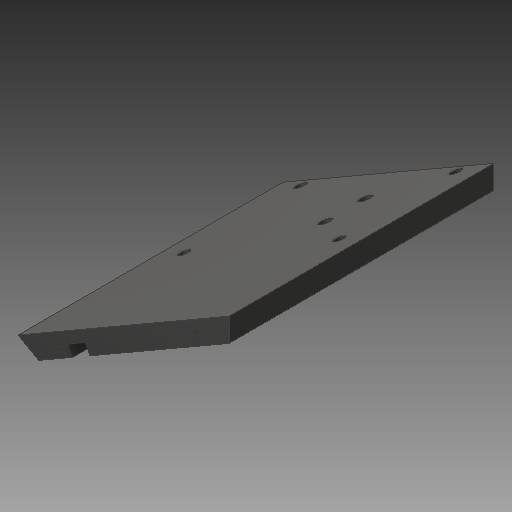
# Autodesk Inventor part: HB02
Saved by Autodesk Inventor 2017 (Build 210142000, 142)
## iProperties
Created: 2019-05-20
Part Number: HB02
Material: Polyethylene, High Density
Document SubType Name: Modeling
Designer: Dell
Density: 0.952 g/cm^3
Appearance: Smooth - Black
Mass: 1765.8 g
Surface Area: 2622.79 cm^2
Volume: 1854.83 cm^3
Author: Dell
Autodesk Inventor part; units mm, degrees
ref_plane "YZ Plane" through (0, 0, 0) normal (1, 0, 0) x (0, 1, 0)
ref_plane "XZ Plane" through (0, 0, 0) normal (0, 1, 0) x (-1, 0, 0)
ref_plane "XY Plane" through (0, 0, 0) normal (0, 0, 1) x (1, 0, 0)
sketch "Sketch1" plane through (0, 0, 0) normal (0, 0, 1) x (1, 0, 0)
  line L0 (262.89, 151.7796) -> (525.78, 0) construction
  line L1 (525.78, 0) -> (525.78, -303.5592) construction
  line L2 (525.78, -303.5592) -> (262.89, -455.3388) construction
  line L3 (262.89, -455.3388) -> (0, -303.5592) construction
  line L4 (0, -303.5592) -> (0, 0) construction
  line L5 (0, 0) -> (262.89, 151.7796)
  line L6 (0, 0) -> (25.4, -14.6647)
  line L7 (25.4, -14.6647) -> (262.89, 122.4502)
  line L8 (262.89, 122.4502) -> (262.89, 151.7796)
  point P0 (262.89, -151.7796)
  dimension "d0" = 525.78
  dimension "d2" = 25.4
  dimension "d3" = 60
  dimension "d4" = 60
  constraints: 18 end point, 1 coincident, 1 parallel, 1 vertical, 13 other
  measures "d0" distance between parallel lines of L1 L4
  measures "d2" distance between parallel lines of L5 L7
  measures "d3" angle of L5 L8
  measures "d4" angle of L5 L6
extrude "Extrusion1" add sketch "Sketch1" along normal blind 330.2
sketch "Sketch8" plane through (0, 0, 0) normal (0, 0, -1) x (-1, 0, 0)
  line L0 (-25.4, -14.6647) -> (-262.89, 122.4502) projected
  line L1 (-67.675, 9.7428) -> (-61.325, 20.7413)
  line L2 (-61.325, 20.7413) -> (-83.322, 33.4413)
  line L3 (-83.322, 33.4413) -> (-89.672, 22.4428)
  line L4 (-67.675, 9.7428) -> (-89.672, 22.4428)
  point P0 (0, 0)
  dimension "d47" = 25.4
  dimension "d48" = 12.7
  dimension "d54" = 48.8149
  constraints: 8 end point, 3 perpendicular, 2 point on line, 1 collinear
  measures "d47" distance of L1.end L2.end
  measures "d48" distance of L1.start L1.end
  measures "d54" distance from line of L1 L0.start
extrude "Extrusion7" cut sketch "Sketch8" against normal blind 25.4
sketch "Sketch9" plane through (0, 0, 330.2) normal (0, 0, 1) x (1, 0, 0)
  line L0 (61.325, 20.7413) -> (67.675, 9.7428) projected
  line L1 (83.322, 33.4413) -> (61.325, 20.7413) projected
  line L2 (89.672, 22.4428) -> (83.322, 33.4413) projected
  line L3 (67.675, 9.7428) -> (89.672, 22.4428) projected
  point P0 (0, 0)
extrude "Extrusion8" cut sketch "Sketch9" against normal blind 185
sketch "Sketch10" plane through (25.4, -14.6647, 0) normal (0.5, -0.8660254, 0) x (0.8660254, 0.5, 0)
  circle A0 centre (25.4, 157.9) radius 2
  circle A1 centre (248.8298, 157.9) radius 2
  line L0 (25.4, 157.9) -> (248.8298, 157.9) construction
  line L1 (288.8945, 330.2) -> (-14.6647, 330.2) projected
  circle A2 centre (25.4, 12.7) radius 2
  circle A3 centre (248.8298, 12.7) radius 2
  line L2 (0, 0) -> (0, 330.2) projected
  line L3 (74.2149, 145.2) -> (48.8149, 145.2) projected
  line L4 (48.8149, 25.4) -> (74.2149, 25.4) projected
  point P0 (-14.6647, 0)
  point P1 (137.1149, 157.9)
  point P2 (137.1149, 330.2)
  dimension "d55" = 4
  dimension "d56" = 4
  dimension "d58" = 4
  dimension "d59" = 4
  dimension "d69" = 25.4
  dimension "d70" = 12.7
  dimension "d71" = 12.7
  constraints: 4 centre point, 3 vertical alignment, 2 end point, 2 midpoint, 1 horizontal, 1 horizontal alignment
  measures "d55" diameter of A0
  measures "d56" diameter of A1
  measures "d58" diameter of A2
  measures "d59" diameter of A3
  measures "d69" distance from line of L2 L0.start
  measures "d70" distance from line of L0.start L3
  measures "d71" distance from line of L4 A2.centre
extrude "Extrusion9" cut sketch "Sketch10" against normal through all
sketch "Sketch11" plane through (0, 0, 330.2) normal (-0.5, 0.8660254, 0) x (0.8660254, 0.5, 0)
  circle A0 centre (263.4945, 172.3) radius 2 projected
  circle A1 centre (40.0647, 172.3) radius 2 projected
  circle A2 centre (40.0647, 317.5) radius 2 projected
  circle A3 centre (263.4945, 317.5) radius 2 projected
  circle A4 centre (263.4945, 172.3) radius 2 projected
  circle A5 centre (263.4945, 172.3) radius 6.5
  circle A6 centre (40.0647, 172.3) radius 6.5
  circle A7 centre (40.0647, 317.5) radius 6.5
  circle A8 centre (263.4945, 317.5) radius 2 projected
  circle A9 centre (263.4945, 317.5) radius 6.5
  point P0 (0, 330.2)
  dimension "d63" = 13
  dimension "d64" = 13
  dimension "d65" = 13
  dimension "d66" = 13
  constraints: 4 centre point, 4 coincident
  measures "d63" diameter of A5
  measures "d64" diameter of A6
  measures "d65" diameter of A7
  measures "d66" diameter of A9
extrude "Extrusion10" cut sketch "Sketch11" against normal blind 12.7 contours A0 | A1 | A2 | A3 | A5 | A6 | A7 | A9
sketch "Sketch12" plane through (0, 0, 330.2) normal (-0.5, 0.8660254, 0) x (0.8660254, 0.5, 0)
  line L0 (288.8945, 330.2) -> (288.8945, 0) construction
  circle A0 centre (188.4945, 269.9) radius 4
  circle A1 centre (188.4945, 219.9) radius 4
  line L1 (88.8796, 330.2) -> (288.8945, 330.2) construction
  line L2 (213.8945, 330.2) -> (163.0945, 330.2) construction
  line L3 (163.0945, 330.2) -> (163.0945, 159.6) construction
  line L4 (163.0945, 159.6) -> (213.8945, 159.6) construction
  line L5 (213.8945, 159.6) -> (213.8945, 330.2) construction
  line L6 (188.4945, 269.9) -> (188.4945, 219.9) construction
  circle A2 centre (263.4945, 172.3) radius 2 construction
  circle A3 centre (263.4945, 317.5) radius 2 construction
  circle A4 centre (263.4945, 172.3) radius 2 construction
  line L7 (263.4945, 172.3) -> (263.4945, 317.5) construction
  point P0 (0, 330.2)
  point P1 (188.4945, 159.6)
  point P2 (188.4945, 244.9)
  point P3 (263.4945, 244.9)
  point P4 (213.8945, 244.9)
  dimension "d72" = 8
  dimension "d73" = 8
  dimension "d74" = 50
  dimension "d75" = 50.8
  dimension "d76" = 75
  constraints: 12 end point, 4 midpoint, 2 centre point, 2 horizontal alignment, 2 parallel, 2 vertical, 1 horizontal, 1 perpendicular, 1 point on line, 1 vertical alignment
  measures "d72" diameter of A1
  measures "d73" diameter of A0
  measures "d74" distance of L6.end L6.start
  measures "d75" distance between parallel lines of L3 L5
  measures "d76" distance between parallel lines of L0 L5
extrude "Extrusion11" cut sketch "Sketch12" against normal through all
sketch "Sketch13" plane through (25.4, -14.6647, 0) normal (0.5, -0.8660254, 0) x (0.8660254, 0.5, 0)
  line L0 (99.6149, 304.8) -> (148.4298, 304.8)
  line L1 (148.4298, 304.8) -> (148.4298, 25.4)
  line L2 (148.4298, 25.4) -> (99.6149, 25.4)
  line L3 (99.6149, 25.4) -> (99.6149, 304.8)
  line L4 (199.2298, 25.4) -> (223.4298, 25.4)
  line L5 (223.4298, 25.4) -> (223.4298, 304.8)
  line L6 (223.4298, 304.8) -> (199.2298, 304.8)
  line L7 (199.2298, 304.8) -> (199.2298, 25.4)
  line L8 (288.8945, 330.2) -> (-14.6647, 330.2) projected
  line L9 (288.8945, 0) -> (-14.6647, 0) projected
  line L10 (148.4298, 110.3) -> (199.2298, 110.3) construction
  circle A0 centre (173.8298, 110.3) radius 4 projected
  line L11 (223.4298, 157.9) -> (274.2298, 157.9)
  line L12 (274.2298, 0) -> (274.2298, 330.2) projected
  circle A1 centre (248.8298, 157.9) radius 2 projected
  line L13 (74.2149, 330.2) -> (74.2149, 145.2) projected
  line L14 (99.6149, 119.8) -> (25.4, 119.8)
  line L15 (25.4, 119.8) -> (25.4, 50.8)
  line L16 (25.4, 50.8) -> (99.6149, 50.8)
  line L17 (99.6149, 50.8) -> (99.6149, 119.8)
  line L18 (74.2149, 145.2) -> (48.8149, 145.2) projected
  line L19 (48.8149, 25.4) -> (74.2149, 25.4) projected
  line L20 (0, 0) -> (0, 330.2) projected
  dimension "d79" = 25.4
  dimension "d80" = 25.4
  dimension "d81" = 25.4
  dimension "d82" = 25.4
  dimension "d83" = 25.4
  dimension "d84" = 25.4
  dimension "d85" = 25.4
  constraints: 28 end point, 6 parallel, 6 point on line, 4 horizontal, 4 perpendicular, 2 coincident, 2 midpoint, 1 horizontal alignment
  measures "d79" distance between parallel lines of L8 L6
  measures "d80" distance between parallel lines of L9 L4
  measures "d81" distance between parallel lines of L13 L3
  measures "d82" distance between parallel lines of L14 L18
  measures "d83" distance between parallel lines of L19 L16
  measures "d84" distance between parallel lines of L20 L15
  measures "d85" distance from line of A0.centre L1
extrude "Extrusion12" cut sketch "Sketch13" against normal blind 19.05 contours L0 L1 L2 L3 | L3 L16 L15 L14 | L7 L6 L5 L4
sketch "Sketch14" plane through (0, 0, 330.2) normal (-0.5, 0.8660254, 0) x (0.8660254, 0.5, 0)
  circle A0 centre (188.4945, 219.9) radius 4 projected
  circle A1 centre (188.4945, 269.9) radius 4 projected
  circle A2 centre (188.4945, 219.9) radius 7.5
  circle A3 centre (188.4945, 269.9) radius 4 projected
  circle A4 centre (188.4945, 269.9) radius 7.5
  point P0 (0, 330.2)
  dimension "d88" = 15
  dimension "d89" = 15
  constraints: 2 centre point, 2 coincident
  measures "d88" diameter of A2
  measures "d89" diameter of A4
extrude "Extrusion13" cut sketch "Sketch14" against normal blind 12.7 contours A0 | A1 | A2 | A4
sketch "Sketch15" plane through (0, 0, 330.2) normal (0, 0, 1) x (1, 0, 0)
  line L0 (0, 0) -> (25.4, -14.6647) projected
  line L1 (12.7, -7.3323) -> (262.89, 137.1149) construction
  line L2 (262.89, 122.4502) -> (262.89, 151.7796) projected
  line L3 (51.1925, 14.8913) -> (224.3975, 114.8913)
  circle A0 centre (51.1925, 14.8913) radius 2
  circle A1 centre (224.3975, 114.8913) radius 2
  point P0 (137.795, 64.8913)
  dimension "d92" = 200
  dimension "d93" = 4
  dimension "d94" = 4
  constraints: 4 end point, 4 midpoint, 2 centre point, 2 coincident, 2 point on line
  measures "d92" distance of L3.end L3.start
  measures "d93" diameter of A0
  measures "d94" diameter of A1
extrude "Extrusion14" cut sketch "Sketch15" against normal blind 38.1
body "Solid1"
